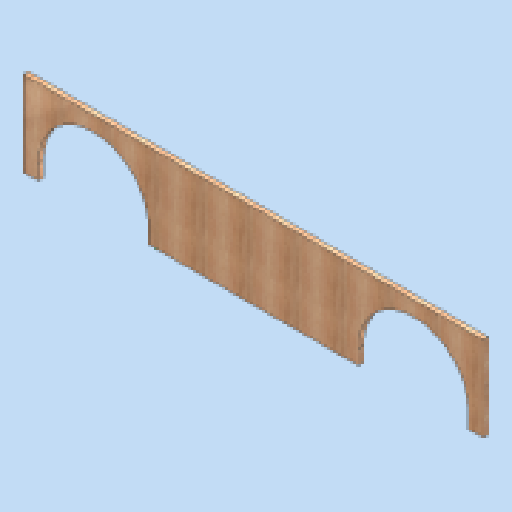
# Autodesk Inventor part: skateboardplank
Saved by Autodesk Inventor 2023 (Build 270158000, 158)
## iProperties
Created: 2026-03-22
Part Number: skateboardplank
Material: Wood (Birch)
Document SubType Name: Modeling
Designer: Nathann
Mass: 27392.9 g
Surface Area: 22398.4 cm^2
Volume: 27392.9 cm^3
Density: 0.55 g/cm^3
Appearance: Birch - Natural Polished
Author: Nathann
Autodesk Inventor part; units mm, degrees
ref_plane "YZ Plane" through (0, 0, 0) normal (1, 0, 0) x (0, 1, 0)
ref_plane "XZ Plane" through (0, 0, 0) normal (0, 1, 0) x (-1, 0, 0)
ref_plane "XY Plane" through (0, 0, 0) normal (0, 0, 1) x (1, 0, 0)
sketch "Sketch1" plane through (0, 0, 0) normal (0, 0, 1) x (1, 0, 0)
  line L0 (-705.0459, 12.4407) -> (1794.9541, 12.4407)
  line L1 (1794.9541, 12.4407) -> (1794.9541, 472.4407)
  line L2 (1794.9541, 472.4407) -> (-705.0459, 472.4407)
  line L3 (-705.0459, 472.4407) -> (-705.0459, 12.4407)
  arc A0 (-25.0459, 92.4407) -> (-625.0459, 92.4407) centre (-325.0459, 92.4407) ccw
  line L4 (-625.0459, 92.4407) -> (-625.0459, 12.4407)
  line L5 (-25.0459, 92.4407) -> (-25.0459, 12.4407)
  line L6 (1760.5221, 12.4407) -> (1110.5221, 12.4407)
  arc A1 (1714.9541, 102.4407) -> (1115.1208, 92.4407) centre (1415.1208, 92.4407) ccw
  line L7 (1115.1208, 92.4407) -> (1115.1208, 12.4407)
  line L8 (1714.9541, 102.4407) -> (1714.9541, 12.4407)
  point P0 (0, 0)
  point P1 (1714.9541, 57.4407)
  point P2 (-625.0459, 52.4407)
  dimension "d0" = 460
  dimension "d1" = 2500
  dimension "d2" = 300
  dimension "d3" = 80
  dimension "d9" = 300
  dimension "d10" = 80
  dimension "d11" = 80
  dimension "d12" = 80
  dimension "d13" = 80
  constraints: 18 end point, 5 point on line, 4 point on circle, 3 perpendicular, 2 centre point, 2 horizontal, 2 midpoint, 2 parallel, 2 tangent
  measures "d0" distance of L2.end L0.start
  measures "d1" distance of L0.start L0.end
  measures "d2" radius of A0
  measures "d3" distance from line of L0 A0.centre
  measures "d9" radius of A1
  measures "d10" distance of L4.start L4.end
  measures "d11" distance from line of L0 A1.centre
  measures "d12" distance from line of point (1714.954, 57.441) L1
  measures "d13" distance from line of L3 point (-625.046, 52.441)
sketch "Sketch3" plane through (0, 0, 0) normal (0, 0, 1) x (1, 0, 0)
  point P0 (0, 0)
extrude "Extrusion1" add sketch "Sketch1" along normal blind 27 contours L3 L2 L1 L0 L8 A1 L7 L5 A0 L4
body "Solid1"
